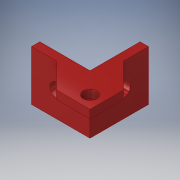
# Autodesk Inventor part: КВ33.044.003 - крепеж дна блока управления
Saved by Autodesk Inventor 2019 (Build 230136000, 136)
## iProperties
Created: 2019-08-10
Part Number: КВ33.044.003 - крепеж дна блока управления
Material: Пластик АБС
Document SubType Name: Modeling
Designer: Петров Иван
Density: 1.06 g/cm^3
Appearance: Красный
Author: Петров Иван
Autodesk Inventor part; units mm, degrees
note: some values were not read from the file. Chosen so that the rebuilt part matches the saved one: second side of "Выдавливание5".
ref_plane "YZ Plane" through (0, 0, 0) normal (1, 0, 0) x (0, 1, 0)
ref_plane "XZ Plane" through (0, 0, 0) normal (0, 1, 0) x (-1, 0, 0)
ref_plane "XY Plane" through (0, 0, 0) normal (0, 0, 1) x (1, 0, 0)
sketch "Эскиз1" plane through (0, 0, 0) normal (0, 0, 1) x (1, 0, 0)
  line L0 (-15, -15) -> (15, -15)
  line L1 (15, -15) -> (15, 15)
  line L2 (15, 15) -> (-15, 15)
  line L3 (-15, 15) -> (-15, -15)
  line L4 (-15, -15) -> (15, 15) construction
  line L5 (15, -15) -> (-15, 15) construction
  line L6 (15, 15) -> (20, 15)
  line L7 (20, 15) -> (20, -15)
  line L8 (20, -15) -> (15, -15)
  line L9 (15, -15) -> (15, 15)
  point P0 (0, 0)
  dimension "d0" = 30
  dimension "d1" = 30
  dimension "d2" = 5
  constraints: 20 end point, 4 parallel, 2 horizontal, 2 midpoint, 2 perpendicular
  measures "d0" distance of L2.end L1.end
  measures "d1" distance of L1.end L0.end
  measures "d2" distance of L7.end L8.end
extrude "Выдавливание1" add sketch "Эскиз1" along normal blind 5
sketch "Эскиз2" plane through (0, 0, 0) normal (0, 0, -1) x (-1, 0, 0)
  line L0 (-20, -15) -> (-20, 15) projected
  line L1 (15, -15) -> (-20, -15) projected
  line L2 (-20, 15) -> (-15, 15)
  line L3 (-15, 15) -> (-15, -15)
  line L4 (-15, -15) -> (-20, -15)
  line L5 (-20, -15) -> (-20, 15)
  point P0 (0, 0)
  dimension "d7" = 5
  constraints: 8 end point, 2 parallel, 1 horizontal, 1 perpendicular, 1 point on line
  measures "d7" distance of L3.end L4.end
extrude "Выдавливание2" add sketch "Эскиз2" along normal blind 30
sketch "Эскиз3" plane through (0, 0, 5) normal (0, 0, 1) x (1, 0, 0)
  line L0 (-15, 15) -> (-15, -15) projected
  line L1 (-15, 0) -> (0, 0)
  circle A0 centre (0, 0) radius 4.1
  dimension "d10" = 15
  dimension "d11" = 8.2
  constraints: 2 end point, 1 centre point, 1 coincident, 1 horizontal, 1 midpoint
  measures "d10" distance of L1.start L1.end
  measures "d11" diameter of A0
sketch "Эскиз4" plane through (20, -15, 5) normal (1, 0, 0) x (0, 0, -1)
  line L0 (35, 30) -> (35, 0) projected
  line L1 (35, 15) -> (20, 15)
  circle A0 centre (20, 15) radius 4.1
  point P0 (5, 15)
  dimension "d12" = 15
  dimension "d13" = 8.2
  constraints: 2 end point, 1 centre point, 1 coincident, 1 horizontal, 1 midpoint
  measures "d12" distance of L1.start L1.end
  measures "d13" diameter of A0
sketch "Эскиз5" plane through (-15, 15, 5) normal (0, 1, 0) x (1, 0, 0)
  line L0 (30, 5) -> (30, 35) projected
  line L1 (30, 5) -> (50, 5)
  line L2 (50, 5) -> (50, -15)
  line L3 (50, -15) -> (30, -15)
  line L4 (30, -15) -> (30, 5)
  point P0 (15, 5)
  dimension "d18" = 20
  dimension "d19" = 20
  constraints: 8 end point, 2 parallel, 1 horizontal, 1 perpendicular
  measures "d18" distance of L2.end L3.end
  measures "d19" distance of L1.end L2.end
extrude "Выдавливание5" add sketch "Эскиз5" against normal blind 5
chamfer "Фаска1" distance 15 angle 45 2 edges at (20, 12.5, 0) (15, 12.5, 5)
chamfer "Фаска2" distance 10 angle 45 2 edges at (17.5, 10, 5) (20, 10, 2.5)
extrude "Выдавливание6" cut sketch "Эскиз3" along normal blind 5 and the other way blind 16.25
extrude "Выдавливание7" cut sketch "Эскиз4" along normal blind 5 and the other way blind 11.5
sketch "Эскиз6" plane through (0, 0, 5) normal (0, 0, 1) x (1, 0, 0)
  circle A0 centre (0, 0) radius 7.5
  dimension "d38" = 15
  constraints: 1 centre point, 1 coincident
  measures "d38" diameter of A0
extrude "Выдавливание8" cut sketch "Эскиз6" along normal blind 10.5
sketch "Эскиз7" plane through (20, -15, -30) normal (1, 0, 0) x (0, 0, -1)
  arc A0 (-19.1, 15) -> (-15, 19.1) centre (-15, 15) ccw projected
  circle A1 centre (-15, 15) radius 7.5
  point P0 (-30, 15)
  point P1 (-15, 10.9)
  dimension "d41" = 15
  constraints: 1 centre point, 1 coincident
  measures "d41" diameter of A1
extrude "Выдавливание9" cut sketch "Эскиз7" along normal blind 10.5
sketch "Эскиз8" plane through (-15, 15, 5) normal (0, 1, 0) x (1, 0, 0)
  line L0 (35, 0) -> (45, -10) projected
  circle A0 centre (42.5, -7.5) radius 4.1
  point P0 (15, 5)
  point P1 (50, -15)
  dimension "d44" = 8.2
  constraints: 1 centre point, 1 point on line
  measures "d44" diameter of A0
extrude "Выдавливание10" cut sketch "Эскиз8" against normal blind 17.25
sketch "Эскиз9" plane through (-15, 10, 5) normal (0, -1, 0) x (1, 0, 0)
  arc A0 (39.2504, 10) -> (39.6009, 4.6009) centre (42.5, 7.5) ccw projected
  circle A1 centre (42.5, 7.5) radius 7.5
  point P0 (15, -5)
  dimension "d47" = 15
  constraints: 1 centre point, 1 coincident
  measures "d47" diameter of A1
extrude "Выдавливание11" cut sketch "Эскиз9" along normal blind 24
